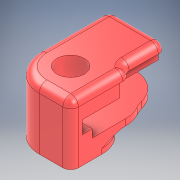
# Autodesk Inventor part: HotBed_Corner_Bracket_Clipped_LN6019
Saved by Autodesk Inventor 2020.3 (Build 243373000, 373)
## iProperties
Created: 2020-04-30
Part Number: HotBed_Corner_Bracket_Clipped_LN6019
Material: ABS Plastic
Document SubType Name: Modeling
Designer: rah75
Density: 1.06 g/cm^3
Appearance: Satin -Light Red
Author: rah75
Autodesk Inventor part; units mm, degrees
ref_plane "YZ Plane" through (0, 0, 0) normal (1, 0, 0) x (0, 1, 0)
ref_plane "XZ Plane" through (0, 0, 0) normal (0, 1, 0) x (-1, 0, 0)
sketch "Sketch1" plane through (0, 0, 0) normal (0, 1, 0) x (-1, 0, 0)
  line L0 (13, -13) -> (-13, -13)
  line L1 (-13, -13) -> (-13, 13)
  line L2 (-13, 13) -> (13, 13)
  line L3 (13, 13) -> (13, -13)
  line L4 (13, -13) -> (-13, 13) construction
  line L5 (-13, -13) -> (13, 13) construction
  line L6 (-209.075, -209.075) -> (10, -209.075)
  line L7 (10, -209.075) -> (10, 10)
  line L8 (10, 10) -> (-209.075, 10)
  line L9 (-209.075, 10) -> (-209.075, -209.075)
  line L10 (-209.075, -209.075) -> (10, 10) construction
  line L11 (10, -209.075) -> (-209.075, 10) construction
  line L12 (-199.5375, -199.5375) -> (0.4625, -199.5375)
  line L13 (0.4625, -199.5375) -> (0.4625, 0.4625)
  line L14 (0.4625, 0.4625) -> (-199.5375, 0.4625)
  line L15 (-199.5375, 0.4625) -> (-199.5375, -199.5375)
  line L16 (-199.5375, -199.5375) -> (0.4625, 0.4625) construction
  line L17 (0.4625, -199.5375) -> (-199.5375, 0.4625) construction
  line L18 (-206.5375, -206.5375) -> (7.4625, -206.5375)
  line L19 (7.4625, -206.5375) -> (7.4625, 7.4625)
  line L20 (7.4625, 7.4625) -> (-206.5375, 7.4625)
  line L21 (-206.5375, 7.4625) -> (-206.5375, -206.5375)
  line L22 (-206.5375, -206.5375) -> (7.4625, 7.4625) construction
  line L23 (7.4625, -206.5375) -> (-206.5375, 7.4625) construction
  line L24 (4.9625, -204.0375) -> (-204.0375, -204.0375) construction
  line L25 (-204.0375, -204.0375) -> (-204.0375, 4.9625) construction
  line L26 (-204.0375, 4.9625) -> (4.9625, 4.9625) construction
  line L27 (4.9625, 4.9625) -> (4.9625, -204.0375) construction
  line L28 (4.9625, -204.0375) -> (-204.0375, 4.9625) construction
  line L29 (-204.0375, -204.0375) -> (4.9625, 4.9625) construction
  circle A0 centre (4.9625, 4.9625) radius 1.875
  point P0 (0, 0)
  point P1 (-99.5375, -99.5375)
  dimension "d0" = 26
  dimension "d1" = 26
  dimension "d2" = 3
  dimension "d3" = 3
  dimension "d4" = 219.075
  dimension "d5" = 200
  dimension "d6" = 200
  dimension "d7" = 214
  dimension "d8" = 214
  dimension "d9" = 209
  dimension "d10" = 209
  dimension "d11" = 3.75
  constraints: 60 end point, 10 midpoint, 10 parallel, 6 perpendicular, 5 horizontal, 1 centre point, 1 coincident
  measures "d0" distance of L1.end L2.end
  measures "d1" distance of L0.end L1.end
  measures "d2" distance between parallel lines of L3 L7
  measures "d3" distance between parallel lines of L2 L8
  measures "d4" distance of L6.start L6.end
  measures "d5" distance of L14.end L13.end
  measures "d6" distance of L13.end L12.end
  measures "d7" distance of L20.end L19.end
  measures "d8" distance of L19.end L18.end
  measures "d9" distance of L25.end L26.end
  measures "d10" distance of L24.end L25.end
  measures "d11" diameter of A0
extrude "Extrusion1" add sketch "Sketch1" along normal mid plane 13 contours L0 L7 L8 L1 L2 L3 | L0 L19 L20 L1 L8 L7 | L0 L13 L14 L1 L20 L19 | L0 L1 L14 L13
ref_plane "Work Plane1" through (0, 4.5, 0) normal (0, 1, 0) x (1, 0, 0)
sketch "Sketch2" plane through (0, 4.5, 0) normal (0, 1, 0) x (1, 0, 0)
  line L0 (-0.4625, -0.4625) -> (199.5375, -0.4625) projected
  line L1 (-0.4625, 199.5375) -> (-0.4625, -0.4625) projected
  line L2 (13, 13) -> (-13, 13) projected
  line L3 (13, -13) -> (13, 13) projected
  point P0 (0, 0)
  point P1 (13, -0.4625)
  point P2 (-0.4625, 13)
extrude "Extrusion2" cut sketch "Sketch2" against normal blind 3.302
sketch "Sketch3" plane through (0, 1.198, 0) normal (0, 1, 0) x (1, 0, 0)
  line L0 (-10, 209.075) -> (-10, -10) projected
  line L1 (-10, -10) -> (209.075, -10) projected
  line L2 (13, 13) -> (-13, 13) projected
  line L3 (13, -13) -> (13, 13) projected
  point P0 (0, 0)
  point P1 (13, -10)
  point P2 (-10, 13)
extrude "Extrusion3" cut sketch "Sketch3" against normal blind 3.302
sketch "Sketch4" plane through (0, -2.104, 0) normal (0, 1, 0) x (1, 0, 0)
  line L0 (-7.4625, 206.5375) -> (-7.4625, -7.4625) projected
  line L1 (-7.4625, -7.4625) -> (206.5375, -7.4625) projected
  line L2 (13, -13) -> (13, 13) projected
  line L3 (13, 13) -> (-13, 13) projected
  point P0 (0, 0)
  point P1 (-7.4625, 13)
  point P2 (13, -7.4625)
extrude "Extrusion4" cut sketch "Sketch4" against normal blind 2.032
sketch "Sketch5" plane through (0, 6.5, 0) normal (0, 1, 0) x (1, 0, 0)
  circle A0 centre (-4.9625, -4.9625) radius 1.875 projected
  circle A1 centre (-4.9625, -4.9625) radius 3.5
  point P0 (0, 0)
  dimension "d21" = 7
  constraints: 1 centre point, 1 coincident
  measures "d21" diameter of A1
extrude "Extrusion5" cut sketch "Sketch5" against normal up to surface (5.302 mm away)
sketch "Sketch6" plane through (0, -6.5, 0) normal (0, -1, 0) x (1, 0, 0)
  line L0 (13, 13) -> (-13, 13) projected
  line L1 (-13, 13) -> (-13, -13) projected
  line L2 (-13, -13) -> (13, -13) projected
  line L3 (13, -13) -> (13, 13) projected
  circle A0 centre (-4.9625, 4.9625) radius 1.875 projected
  line L4 (-4.9625, 8.1379) -> (-2.2125, 6.5502)
  line L5 (-2.2125, 6.5502) -> (-2.2125, 3.3748)
  line L6 (-2.2125, 3.3748) -> (-4.9625, 1.7871)
  line L7 (-4.9625, 1.7871) -> (-7.7125, 3.3748)
  line L8 (-7.7125, 3.3748) -> (-7.7125, 6.5502)
  line L9 (-7.7125, 6.5502) -> (-4.9625, 8.1379)
  point P0 (0, 0)
  dimension "d24" = 5.5
  constraints: 12 end point, 1 coincident, 1 vertical, 13 other
  measures "d24" distance between parallel lines of L5 L8
extrude "Extrusion6" cut sketch "Sketch6" against normal blind 1 contours L4 L5 L6 L7 L8 L9
sketch "Sketch7" plane through (0, -6.5, 0) normal (0, -1, 0) x (1, 0, 0)
  circle A0 centre (-4.9625, 4.9625) radius 1.875 projected
  circle A1 centre (-4.9625, 4.9625) radius 8.0375
  line L0 (-7.7125, 3.3748) -> (-7.7125, 6.5502) projected
  line L1 (-4.9625, 1.7871) -> (-7.7125, 3.3748) projected
  line L2 (-2.2125, 3.3748) -> (-4.9625, 1.7871) projected
  line L3 (-2.2125, 6.5502) -> (-2.2125, 3.3748) projected
  line L4 (-4.9625, 8.1379) -> (-2.2125, 6.5502) projected
  line L5 (-7.7125, 6.5502) -> (-4.9625, 8.1379) projected
  circle A2 centre (-4.9625, 4.9625) radius 1.875 projected
  line L6 (-13, 13) -> (-13, -13) projected
  point P0 (0, 0)
  constraints: 1 centre point, 1 coincident, 1 tangent
extrude "Extrusion7" add sketch "Sketch7" along normal blind 1 contours A1
sketch "Sketch8" plane through (-4.9625, -7.5, 4.9625) normal (0, -1, 0) x (1, 0, 0)
  circle A0 centre (0, 0) radius 8.0375 projected
  line L0 (-2.75, -1.5877) -> (-2.75, 1.5877) projected
  line L1 (-2.75, 1.5877) -> (0, 3.1754) projected
  line L2 (0, 3.1754) -> (2.75, 1.5877) projected
  line L3 (2.75, 1.5877) -> (2.75, -1.5877) projected
  line L4 (2.75, -1.5877) -> (0, -3.1754) projected
  line L5 (0, -3.1754) -> (-2.75, -1.5877) projected
  circle A1 centre (0, 0) radius 7.0375
  point P0 (4.9625, -4.9625)
  dimension "d30" = 1
  constraints: 1 centre point
  measures "d30" radial gap between concentric circles of A0 A1
extrude "Extrusion8" add sketch "Sketch8" along normal blind 1.5 contours A0
sketch "Sketch9" plane through (-4.9625, -9, 4.9625) normal (0, -1, 0) x (1, 0, 0)
  arc A0 (-8.0375, 0) -> (0, 8.0375) centre (0, 0) ccw projected
  line L0 (17.9625, 8.0375) -> (0, 8.0375) projected
  line L1 (-8.0375, 8.0375) -> (-8.0375, 0) projected
  line L2 (-8.0375, -17.9625) -> (17.9625, -17.9625) projected
  line L3 (17.9625, -17.9625) -> (17.9625, 8.0375) projected
  line L4 (8.0375, 8.0375) -> (-8.0375, 8.0375)
  line L5 (-8.0375, 8.0375) -> (-8.0375, -8.0375)
  line L6 (-8.0375, -8.0375) -> (8.0375, -8.0375)
  line L7 (8.0375, -8.0375) -> (8.0375, 8.0375)
  line L8 (8.0375, 8.0375) -> (-8.0375, -8.0375) construction
  line L9 (-8.0375, 8.0375) -> (8.0375, -8.0375) construction
  circle A1 centre (0, 0) radius 8.0375 projected
  line L10 (-8.0375, 0) -> (-8.0375, -17.9625) projected
  arc A2 (0, 8.0375) -> (-8.0375, 0) centre (0, 0) ccw projected
  line L11 (0, 8.0375) -> (-8.0375, 8.0375) projected
  point P0 (4.9625, -4.9625)
  point P1 (-8.0375, 0)
  point P2 (8, 0)
  point P3 (0, 8)
  point P4 (0, -8.0375)
  point P5 (-8, -0.7755)
  point P6 (0, 8.0375)
  point P7 (8, 0.7755)
  point P8 (8.0375, 0)
  point P9 (0.7755, -8)
  point P10 (-0.7755, -8)
  point P11 (0, 8.0375)
  point P12 (0, 8.0375)
  point P13 (0, 8.0375)
  point P14 (0, 8.0375)
  constraints: 12 end point, 2 midpoint, 2 parallel, 2 tangent, 1 horizontal, 1 perpendicular
extrude "Extrusion9" add sketch "Sketch9" against normal up to surface (2.5 mm away) contours A0 L0 L7 | A1 L1 L4 | L6 L5 A0
sketch "Sketch10" plane through (0, 6.5, 0) normal (0, 1, 0) x (1, 0, 0)
  line L0 (13, 13) -> (-0.4625, 13) projected
  line L1 (13, -0.4625) -> (13, 13) projected
  line L2 (-0.4625, -0.4625) -> (13, -0.4625) projected
  line L3 (-0.4625, 13) -> (-0.4625, -0.4625) projected
  line L4 (13, 13) -> (1.5375, 13)
  line L5 (1.5375, 13) -> (1.5375, 1.5375)
  line L6 (1.5375, 1.5375) -> (13, 1.5375)
  line L7 (13, 1.5375) -> (13, 13)
  point P0 (0, 0)
  point P1 (1.5375, 13)
  dimension "d35" = 2
  dimension "d36" = 2
  constraints: 8 end point, 2 parallel, 1 horizontal, 1 perpendicular
  measures "d35" distance between parallel lines of L5 L3
  measures "d36" distance between parallel lines of L2 L6
extrude "Extrusion10" cut sketch "Sketch10" against normal blind 21 contours L1 L6 L5 L0
fillet "Fillet1" radius 8 4 edges at (1.5375, -5.318, -13) (13, -5.318, -1.5375) (1.5375, -5.318, -1.5375) (-13, -1.25, 13)
fillet "Fillet2" radius 2 7 edges at (13, 0, 13) (1.5375, 5.5, -1.5375) (13, 5.5, -1.5375) (1.5375, 5.5, -13) (-13, 0, -13) (3.075, -7.75, 13) (-13, -7.75, -3.075)
sketch "Sketch11" plane through (0, -6.5, 0) normal (0, -1, 0) x (1, 0, 0)
  arc A0 (-13, -11) -> (-11, -13) centre (-11, -11) ccw projected
  line L0 (-11, -13) -> (-6.4625, -13) projected
  arc A1 (-6.4625, -13) -> (1.2804, -7.0117) centre (-6.4625, -5) ccw projected
  arc A2 (7.0117, -1.2804) -> (1.2804, -7.0117) centre (9.0234, -9.0234) ccw projected
  arc A3 (7.0117, -1.2804) -> (13, 6.4625) centre (5, 6.4625) ccw projected
  line L1 (13, 6.4625) -> (13, 11) projected
  arc A4 (13, 11) -> (11, 13) centre (11, 11) ccw projected
  line L2 (3.075, 11) -> (3.075, 4.9625) projected
  arc A5 (-4.9625, -3.075) -> (3.075, 4.9625) centre (-4.9625, 4.9625) ccw projected
  line L3 (-4.9625, -3.075) -> (-11, -3.075) projected
  line L4 (11, 13) -> (1.075, 13) projected
  arc A6 (3.075, 11) -> (1.075, 13) centre (1.075, 11) ccw projected
  arc A7 (-13, -1.075) -> (-11, -3.075) centre (-11, -1.075) ccw projected
  line L5 (-13, -1.075) -> (-13, -11) projected
  point P0 (0, 0)
extrude "Extrusion11" cut sketch "Sketch11" against normal blind 0.75
fillet "Fillet4" radius 2 5 edges at (3.075, -5.75, 7.9813) (2.4892, -5.75, 12.4142) (-7.9813, -5.75, -3.075) (-12.4142, -5.75, -2.4892) (0.7209, -5.75, -0.7209)
sketch "Sketch12" plane through (0, -5.75, 0) normal (0, -1, 0) x (1, 0, 0)
  line L0 (3.075, 4.9625) -> (3.075, 11) projected
  arc A0 (3.075, 11) -> (1.075, 13) centre (1.075, 11) ccw projected
  line L1 (3.075, 11) -> (3.075, 4.9625) projected
  line L2 (3.075, 4.9625) -> (3.075, -5.656)
  line L3 (3.075, -5.656) -> (13, -5.656)
  line L4 (13, -5.656) -> (13, 13)
  line L5 (13, 13) -> (1.075, 13)
  line L6 (13, 11) -> (13, 6.4625) projected
  point P0 (0, 0)
  dimension "d45" = 18.656
  constraints: 8 end point, 3 perpendicular, 1 collinear, 1 vertical
  measures "d45" distance of L3.end L4.end
extrude "Extrusion12" cut sketch "Sketch12" along normal mid plane 32.75
fillet "Fillet5" radius 8 1 edges at (3.075, -4.943, -3.6739)
fillet "Fillet6" radius 2 1 edges at (3.075, 5.5, -1.5917)
fillet "Fillet7" radius 2 12 edges at (2.8726, 6.5, -1.2621) (1.7399, 6.5, -2.6607) (1.5375, 6.5, -4.8696) (1.5375, 6.5, -8.6009) (0.9517, 6.5, -12.4142) (-5.7313, 6.5, -13) (-12.4142, 6.5, -12.4142) (-13, 6.5, -3) (-10.6569, 6.5, 10.6569) (-1.9625, 6.5, 13) (2.4892, 6.5, 12.4142) (3.075, 6.5, 5.3073)
equation "\"d36\" = d35"
body "Solid1"
